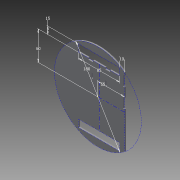
# Autodesk Inventor part: BasePlate
Saved by Autodesk Inventor 2015 (Build 190159000, 159)
## iProperties
Created: 2014-07-26
Part Number: BasePlate
Material: Generic
Document SubType Name: Modeling
Designer: karl
Density: 1 g/cm^3
Appearance: Default
Author: karl
Autodesk Inventor part; units mm, degrees
ref_plane "YZ Plane" through (0, 0, 0) normal (1, 0, 0) x (0, 1, 0)
ref_plane "XZ Plane" through (0, 0, 0) normal (0, 1, 0) x (-1, 0, 0)
ref_plane "XY Plane" through (0, 0, 0) normal (0, 0, 1) x (1, 0, 0)
sketch "Sketch1" plane through (0, 0, 0) normal (0, 1, 0) x (-1, 0, 0)
  circle A0 centre (0, 0) radius 90 construction
  line L0 (-55, 71.239) -> (-55, -71.239) construction
  line L1 (-45, 75) -> (40, 75) construction
  line L2 (40, 75) -> (40, 60) construction
  line L3 (40, 60) -> (-45, 60) construction
  line L4 (-45, 60) -> (-45, 75) construction
  line L5 (-55, 0) -> (0, 0) construction
  circle A1 centre (0, 0) radius 90 construction
  line L6 (-45, -75) -> (40, -75) construction
  line L7 (40, -75) -> (40, -60) construction
  line L8 (40, -60) -> (-45, -60) construction
  line L9 (-45, -60) -> (-45, -75) construction
  line L10 (-2.5, 60) -> (-2.5, -60) construction
  dimension "d0" = 180
  dimension "d1" = 55
  dimension "d2" = 85
  dimension "d3" = 60
  dimension "d4" = 10
  dimension "d5" = 15
  constraints: 22 end point, 4 symmetric about line, 3 midpoint, 2 centre point, 2 horizontal, 2 parallel, 2 point on circle, 1 coincident, 1 perpendicular, 1 vertical, 1 other
  measures "d0" diameter of A0
  measures "d1" distance from line of point (0, 0) L0
  measures "d2" distance of L2.end L3.end
  measures "d3" distance from line of point (0, 0) L3
  measures "d4" distance between parallel lines of L0 L4
  measures "d5" distance between parallel lines of L3 L1
sketch "Sketch2" plane through (0, 0, 0) normal (0, 1, 0) x (-1, 0, 0)
  circle A0 centre (0, 0) radius 90
  line L0 (-55, -71.239) -> (-55, 71.239)
  dimension "d6" = 180
  dimension "d7" = 55
  constraints: 2 end point, 2 point on circle, 1 centre point, 1 coincident, 1 vertical
  measures "d6" diameter of A0
  measures "d7" distance from line of point (0, 0) L0
extrude "Extrusion1" add sketch "Sketch2" along normal blind 3 contours A0 L0 picked at (-6.6667, 0)
sketch "Sketch3" plane through (0, 3, 0) normal (0, 1, 0) x (1, 0, 0)
  line L0 (-40, -60) -> (45, -60) construction
  line L1 (45, -60) -> (45, -75) construction
  line L2 (-40, -75) -> (-40, -60) construction
  line L3 (45, -75) -> (-40, -75) construction
  line L4 (45, -60) -> (-40, -60)
  line L5 (-40, -60) -> (-40, -75)
  line L6 (-40, -75) -> (45, -75)
  line L7 (45, -75) -> (45, -60)
  point P0 (0, 0)
  constraints: 8 end point, 2 parallel, 1 horizontal, 1 perpendicular
extrude "Extrusion2" cut sketch "Sketch3" against normal blind 3
mirror "Mirror1" about plane through (0, 0, 0) normal (0, 0, 1) of "Extrusion2"
sketch "Sketch4" plane through (0, 3, 0) normal (0, 1, 0) x (1, 0, 0)
  line L0 (2.5, -60) -> (2.5, 60)
  line L1 (15, -5) -> (-10, -5) construction
  line L2 (-10, -5) -> (-10, -57) construction
  line L3 (-10, -57) -> (15, -57) construction
  line L4 (15, -57) -> (15, -5) construction
  line L5 (15, -5) -> (-10, -57) construction
  line L6 (-10, -5) -> (15, -57) construction
  line L7 (-40, -60) -> (45, -60) construction
  line L8 (45, 60) -> (-40, 60) construction
  line L9 (45, -60) -> (-40, -60) projected
  line L10 (-10, -60) -> (-20, -60)
  line L11 (-20, -60) -> (-20, -57)
  line L12 (-20, -57) -> (-10, -57)
  line L13 (-10, -57) -> (-10, -60)
  line L14 (15, -57) -> (25, -57)
  line L15 (25, -57) -> (25, -60)
  line L16 (25, -60) -> (15, -60)
  line L17 (15, -60) -> (15, -57)
  line L18 (-10, -37) -> (-13, -37)
  line L19 (-13, -37) -> (-13, -27)
  line L20 (-13, -27) -> (-10, -27)
  line L21 (-10, -27) -> (-10, -37)
  line L22 (15, -37) -> (18, -37)
  line L23 (18, -37) -> (18, -27)
  line L24 (18, -27) -> (15, -27)
  line L25 (15, -27) -> (15, -37)
  point P0 (0, 0)
  point P1 (2.5, -31)
  dimension "d12" = 25
  dimension "d13" = 52
  dimension "d14" = 3
  dimension "d15" = 10
  dimension "d16" = 10
  dimension "d17" = 3
  dimension "d18" = 10
  dimension "d19" = 20
  dimension "d20" = 3
  dimension "d21" = 10
  constraints: 46 end point, 10 parallel, 5 horizontal, 5 perpendicular, 5 point on line, 4 midpoint, 3 collinear
  measures "d12" distance of L3.end L2.end
  measures "d13" distance of L2.end L1.end
  measures "d14" distance between parallel lines of L7 L3
  measures "d15" distance of L11.end L12.end
  measures "d16" distance of L15.end L16.end
  measures "d17" distance of L19.end L20.end
  measures "d18" distance of L18.end L19.end
  measures "d19" distance between parallel lines of L12 L18
  measures "d20" distance of L24.end L23.end
  measures "d21" distance of L23.end L22.end
extrude "Extrusion3" cut sketch "Sketch4" against normal blind 3
sketch "Sketch5" plane through (0, 3, 0) normal (0, 1, 0) x (1, 0, 0)
  line L0 (55, -71.239) -> (55, 71.239) projected
  line L1 (55, -65) -> (52, -65)
  line L2 (52, -65) -> (52, -45)
  line L3 (52, -45) -> (55, -45)
  line L4 (55, -45) -> (55, -65)
  line L5 (55, -25) -> (52, -25)
  line L6 (52, -25) -> (52, -5)
  line L7 (52, -5) -> (55, -5)
  line L8 (55, -5) -> (55, -25)
  point P0 (0, 0)
  dimension "d24" = 3
  dimension "d25" = 20
  dimension "d26" = 20
  dimension "d27" = 20
  dimension "d28" = 5
  constraints: 16 end point, 4 parallel, 3 point on line, 2 horizontal, 2 perpendicular
  measures "d24" distance of L2.end L3.end
  measures "d25" distance of L1.end L2.end
  measures "d26" distance of L5.end L6.end
  measures "d27" distance between parallel lines of L3 L5
  measures "d28" distance from line of point (0, 0) L7
extrude "Extrusion4" cut sketch "Sketch5" against normal blind 3
body "Solid1"
